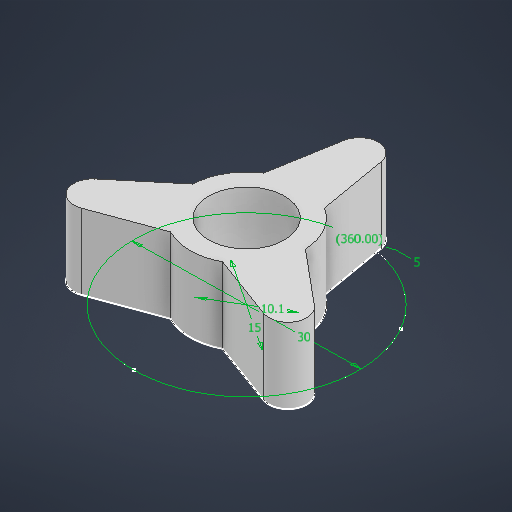
# Autodesk Inventor part: Turret_Holder
Saved by Autodesk Inventor 2026.2 (Build 302298000, 298)
## iProperties
Created: 2025-12-28
Part Number: Turret_Holder
Material: Generic
Document SubType Name: Modeling
Designer: Cobble
Density: 1 g/cm^3
Appearance: Default
Author: Cobble
Autodesk Inventor part; units mm, degrees
ref_plane "YZ Plane" through (0, 0, 0) normal (1, 0, 0) x (0, 1, 0)
ref_plane "XZ Plane" through (0, 0, 0) normal (0, 1, 0) x (-1, 0, 0)
ref_plane "XY Plane" through (0, 0, 0) normal (0, 0, 1) x (1, 0, 0)
sketch "Sketch1" plane through (0, 0, 0) normal (0, 0, 1) x (1, 0, 0)
  circle A0 centre (0, 0) radius 5.05
  circle A1 centre (0, 0) radius 15 construction
  line L0 (0, 0) -> (0, 15)
  circle A2 centre (0, 15) radius 2.5
  line L1 (2.4636, 15.425) -> (4.9765, 0.8585)
  line L2 (-4.9765, 0.8585) -> (-2.4636, 15.425)
  line L3 (0, 0) -> (-12.9904, -7.5)
  circle A3 centre (-12.9904, -7.5) radius 2.5
  line L4 (-14.5902, -5.579) -> (-3.2317, 3.8805)
  line L5 (1.7448, -4.739) -> (-12.1266, -9.846)
  line L6 (0, 0) -> (12.9904, -7.5)
  circle A4 centre (12.9904, -7.5) radius 2.5
  line L7 (12.1266, -9.846) -> (-1.7448, -4.739)
  line L8 (3.2317, 3.8805) -> (14.5902, -5.579)
  circle A5 centre (0, 0) radius 7.5
  point P0 (0, -15)
  point P1 (12.9904, 7.5)
  point P2 (-12.9904, 7.5)
  point P3 (-4.0338, 6.3228)
  point P4 (-3.4588, -6.6548)
  point P5 (3.4588, -6.6548)
  point P6 (4.0338, 6.3228)
  point P7 (7.4926, 0.332)
  point P8 (4.6604, 2.6907)
  point P9 (-7.4926, 0.332)
  point P10 (-4.6604, 2.6907)
  point P11 (0, -5.3814)
  dimension "d0" = 10.1
  dimension "d1" = 30
  dimension "d2" = 5
  dimension "d5" = 360
  dimension "d7" = 15
  constraints: 18 end point, 10 point on circle, 6 centre point, 6 coincident, 4 tangent, 3 point on line, 1 vertical, 37 other
  measures "d0" diameter of A0
  measures "d1" diameter of A1
  measures "d2" diameter of A2
  measures "d7" diameter of A5
extrude "Extrusion1" add sketch "Sketch1" along normal blind 10 contours A0 L1 L8 A5 L6 | A0 L8 L1 | L6 A5 L7 L5 A0 | A0 L0 A5 L1 L8 | L1 A5 L8 | L5 L7 A0 | A5 L8 A4 L6 | L6 A4 L7 A5 | A0 L4 L2 A5 L0 | A5 L0 A2 L1 | L7 L5 A5 L3 A0 | L7 A5 L5 | L3 A5 L4 L2 A0 | A4 | A0 L2 L4 | A5 L2 A2 L0 | A2 | L5 A3 L3 A5 | L3 A3 L4 A5 | L4 A5 L2 | A3
extrude "Extrusion2" add sketch "Sketch1" along normal blind 2 contours A0 L6 L0 | A0 L3 L6 | L3 A0 L0
body "Solid1"
